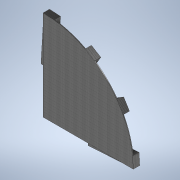
# Autodesk Inventor part: Side Shield
Saved by Autodesk Inventor 2020 (Build 240168000, 168)
## iProperties
Created: 2021-01-17
Part Number: Side Shield
Material: Generic
Document SubType Name: Modeling
Designer: magda
Density: 1 g/cm^3
Appearance: Engine Turned
Author: magda
Autodesk Inventor part; units mm, degrees
ref_plane "YZ Plane" through (0, 0, 0) normal (1, 0, 0) x (0, 1, 0)
ref_plane "XZ Plane" through (0, 0, 0) normal (0, 1, 0) x (-1, 0, 0)
ref_plane "XY Plane" through (0, 0, 0) normal (0, 0, 1) x (1, 0, 0)
sketch "Sketch1" plane through (0, 0, 0) normal (0, 0, 1) x (1, 0, 0)
  line L0 (0, 0) -> (0, 200.025)
  line L1 (0, 0) -> (200.025, 0)
  arc A0 (200.025, 0) -> (0, 200.025) centre (0, 0) ccw
  line L2 (0, 200.025) -> (0, 209.55)
  line L3 (200.025, 0) -> (209.55, 0)
  arc A1 (209.55, 0) -> (0, 209.55) centre (0, 0) ccw
  line L4 (0, 0) -> (25.5377, 207.988)
  line L5 (0, 0) -> (207.988, 25.5377)
  line L6 (0, 0) -> (185.5908, 97.2998)
  line L7 (0, 0) -> (97.2998, 185.5908)
  line L8 (0, 0) -> (119.1924, 172.3496)
  line L9 (0, 0) -> (172.3496, 119.1924)
  line L10 (92.8771, 177.1549) -> (113.7745, 164.5155)
  line L11 (113.7745, 164.5155) -> (61.1935, 77.5799)
  line L12 (61.1935, 77.5799) -> (40.2961, 90.2193)
  line L13 (40.2961, 90.2193) -> (92.8771, 177.1549)
  line L14 (0, 200.025) -> (24.3769, 198.534)
  line L15 (24.3769, 198.534) -> (18.1744, 97.1235)
  line L16 (18.1744, 97.1235) -> (-6.2025, 98.6145)
  line L17 (-6.2025, 98.6145) -> (0, 200.025)
  line L18 (164.5155, 113.7745) -> (177.1549, 92.8771)
  line L19 (177.1549, 92.8771) -> (90.2193, 40.2961)
  line L20 (90.2193, 40.2961) -> (77.5799, 61.1935)
  line L21 (77.5799, 61.1935) -> (164.5155, 113.7745)
  line L22 (198.534, 24.3769) -> (200.025, 0)
  line L23 (200.025, 0) -> (98.6145, -6.2025)
  line L24 (98.6145, -6.2025) -> (97.1235, 18.1744)
  line L25 (97.1235, 18.1744) -> (198.534, 24.3769)
  point P0 (0, 204.7875)
  dimension "d2" = 200.025
  dimension "d3" = 200.025
  dimension "d4" = 200.025
  dimension "d5" = 209.55
  dimension "d6" = 209.55
  dimension "d7" = 7
  dimension "d8" = 7
  dimension "d9" = 27.667
  dimension "d10" = 27.667
  dimension "d11" = 7
  dimension "d12" = 7
  dimension "d13" = 101.6
  dimension "d14" = 101.6
  dimension "d15" = 101.6
  dimension "d16" = 101.6
  constraints: 52 end point, 16 point on circle, 8 parallel, 6 point on line, 4 perpendicular, 2 centre point, 1 concentric, 1 horizontal, 1 midpoint, 1 vertical
  measures "d2" distance of L0.start L0.end
  measures "d3" distance of L0.start L1.end
  measures "d4" radius of A0
  measures "d5" distance from line of L1 L2.end
  measures "d6" distance from line of L0 L3.end
  measures "d7" angle of L4 L0
  measures "d8" angle of L1 L5
  measures "d9" angle of L6 L1
  measures "d10" angle of L7 L0
  measures "d11" angle of L8 L7
  measures "d12" angle of L6 L9
  measures "d13" distance of L10.end L11.end
  measures "d14" distance of L14.end L15.end
  measures "d15" distance of L18.end L19.end
  measures "d16" distance of L1.end L23.end
extrude "Extrusion1" add sketch "Sketch1" along normal blind 1.5875 contours L5 L24 L1 | L0 L16 L4 | L6 L20 L19 A0 L25 L24 L5 | L9 L20 L6 | L4 L16 L15 A0 L13 L12 L7 | L7 L12 L8 | L8 L12 L11 A0 L21 L20 L9 | L0 L14 L4 L16 | L24 L5 L22 L1 | L4 L15 L16 | L24 L25 L5 | L20 L9 L18 L6 | L6 L19 L20 | L12 L13 L7 | L7 L10 L8 L12 | L8 L11 L12 | L20 L21 L9
extrude "Extrusion2" add sketch "Sketch1" against normal blind 12.7 contours L16 L17 L0 | L0 L14 L4 L16 | L24 L5 L22 L1 | L1 L23 L24 | L4 L15 L16 | L24 L25 L5 | L20 L9 L18 L6 | L6 L19 L20 | L12 L13 L7 | L7 L10 L8 L12 | L8 L11 L12 | L20 L21 L9
body "Solid1"
